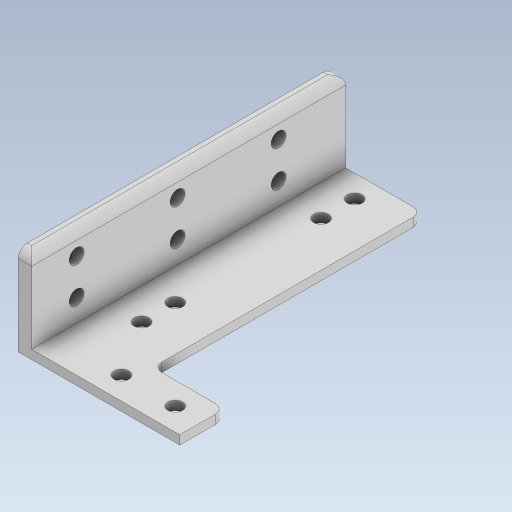
# Autodesk Inventor part: Holder Conveyor Kanan
Saved by Autodesk Inventor 2023.5 (Build 275446000, 446)
## iProperties
Created: 2025-10-12
Part Number: Holder Conveyor Kanan
Material: Generic
Document SubType Name: Modeling
Designer: Guntur
Density: 1 g/cm^3
Appearance: Default
Author: Guntur
## iProperties of the stored document Holder Conveyor Kanan_3DPrint.ipt
Created: 2025-10-20
Part Number: Holder Conveyor Kanan_3DPrint
Material: Generic
Document SubType Name: Modeling
Designer: Guntur
Density: 1 g/cm^3
Appearance: Default
Author: Guntur
Autodesk Inventor part; units mm, degrees
ref_plane "YZ Plane" through (0, 0, 0) normal (1, 0, 0) x (0, 1, 0)
ref_plane "XZ Plane" through (0, 0, 0) normal (0, 1, 0) x (-1, 0, 0)
ref_plane "XY Plane" through (0, 0, 0) normal (0, 0, 1) x (1, 0, 0)
sketch "Sketch1" plane through (0, 0, 0) normal (0, 1, 0) x (-1, 0, 0)
  circle A0 centre (-18, -5) radius 1.65
  line L0 (0, -10) -> (-36, -10)
  line L1 (-36, 0) -> (0, 0)
  line L2 (0, -10) -> (-36, 0) construction
  line L3 (-36, -10) -> (0, 0) construction
  circle A1 centre (-10, -17.5) radius 1.65
  line L4 (0, 0) -> (0, -10)
  line L5 (-20, 0) -> (-20, -35)
  line L6 (0, -35) -> (0, 0)
  line L7 (0, -35) -> (-20, 0) construction
  line L8 (-20, -35) -> (0, 0) construction
  line L9 (-3, 0) -> (-3, -65)
  line L10 (0, -65) -> (0, 0)
  line L11 (0, 0) -> (-3, 0)
  line L12 (0, 0) -> (-20, 0)
  circle A2 centre (-10, -57.5) radius 1.65
  line L13 (-20, -35) -> (0, -35)
  line L14 (-20, -35) -> (0, -35)
  line L15 (0, -65) -> (-20, -65)
  line L16 (-20, -65) -> (-20, -35)
  line L17 (-3, -65) -> (0, -65)
  line L18 (0, -35) -> (0, -65)
  circle A3 centre (-30, -5) radius 1.65
  line L19 (-36, -10) -> (-36, 0)
  circle A4 centre (-10, -25) radius 1.65
  circle A5 centre (-10, -65) radius 1.65
  line L20 (0, -65) -> (-20, -65)
  line L21 (-20, -65) -> (-20, -70)
  line L22 (-20, -70) -> (0, -70)
  line L23 (0, -70) -> (0, -65)
  line L24 (-3, -65) -> (-3, -70)
  point P0 (0, 0)
  point P1 (-20, -10)
  point P2 (-18, -5)
  point P3 (-11.65, -65)
  point P4 (-8.35, -65)
  dimension "d22" = 3.3
  dimension "d23" = 20
  dimension "d24" = 3.3
  dimension "d25" = 40
  dimension "d26" = 5
  constraints: 50 end point, 6 centre point, 3 point on line, 2 parallel, 2 perpendicular, 1 coincident, 1 horizontal, 1 midpoint
  measures "d22" diameter of A4
  measures "d23" vertical distance of point (-18, -5) A4.centre
  measures "d24" diameter of A5
  measures "d25" distance of A4.centre A5.centre
  measures "d26" distance of L21.end L20.end
extrude "Extrusion1" add sketch "Sketch1" along normal blind 2 contours L9 L13 L5 L0 | L0 L5 L1 L9 | L0 L19 L1 L5 | L9 L15 A5 L16 L13 | L23 L22 L24 L15 | L24 L22 L21 L15 A5
extrude "Extrusion2" add sketch "Sketch1" along normal blind 20 contours L6 L13 L9 L0 | L0 L9 L1 L4 | L10 L15 L9 L13 | L23 L22 L24 L15
sketch "Sketch3" plane through (0, 0, -70) normal (-1, 0, 0) x (0, 0, 1)
  circle A0 centre (60, 15) radius 1.65
  line L0 (0, 20) -> (70, 20) projected
  line L1 (70, 0) -> (70, 20) projected
  circle A1 centre (37.5, 15) radius 1.65
  line L2 (37.5, 15) -> (37.5, 0)
  circle A2 centre (60, 7) radius 1.65
  circle A3 centre (15, 15) radius 1.65
  circle A4 centre (15, 7) radius 1.65
  circle A5 centre (37.5, 7) radius 1.65
  dimension "d27" = 3.3
  dimension "d28" = 5
  dimension "d29" = 10
  dimension "d30" = 3.3
  dimension "d31" = 22.5
  dimension "d32" = 3.3
  dimension "d33" = 8
  dimension "d34" = 3.3
  constraints: 6 centre point, 2 end point, 2 symmetric about line, 1 point on line, 1 vertical, 2 other
  measures "d27" diameter of A0
  measures "d28" distance from line of L0 A0.centre
  measures "d29" distance from line of L1 A0.centre
  measures "d30" diameter of A1
  measures "d31" distance of A0.centre L2.start
  measures "d32" diameter of A2
  measures "d33" distance of A0.centre A2.centre
  measures "d34" diameter of A5
extrude "Extrusion4" cut sketch "Sketch3" against normal blind 20
fillet "Fillet1" radius 2 6 edges at (36, 1, -10) (20, 1, -10) (20, 1, -70) (3, 20, -35) (1.5, 20, 0) (1.5, 20, -70)
body "Solid1"
